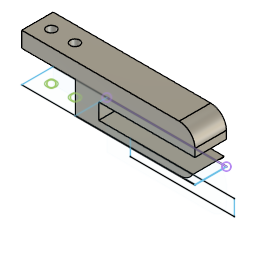
Boczniki (Autodesk Fusion 360 design; units mm, degrees)
part number: 2025-11-04-18-30-34-316
Autodesk Fusion 360 part; units mm, degrees
sketch "Szkic1" plane through (0, 0, 0) normal (0, 0, 1) x (1, 0, 0)
  line L0 (1, 16) -> (111, 16)
  line L1 (111, 16) -> (111, -4)
  line L2 (111, -4) -> (1, -4)
  line L3 (1, -4) -> (1, 16)
  line L4 (35.0688, 16) -> (111, 16)
  line L5 (111, 16) -> (111, -4)
  line L6 (111, -4) -> (35.0688, -4)
  line L7 (35.0688, -4) -> (35.0688, 16)
  circle A0 centre (9.8569, 6) radius 3
  circle A1 centre (24.8569, 6) radius 3
  dimension "d3" = 20
  dimension "d4" = 110
  dimension "d5" = 6
  dimension "d6" = 10
  dimension "d7" = 6
  constraint horizontal L0
  constraint vertical L1
  constraint horizontal L2
  constraint vertical L3
  constraint horizontal L4
  constraint vertical L5
  constraint horizontal L6
  constraint vertical L7
  constraint coincident L0 L4.start
  measures "d3" distance of L0.end L1.end
  measures "d4" distance of L0.start L0.end
  measures "d5" diameter of A0
  measures "d6" distance of L0 A0.centre
  measures "d7" diameter of A1
extrude "Wyciągnięcie proste1" add sketch "Szkic1" against normal blind 30 contours L0 L1 L2 L4 L5 L6 L7
extrude "Wyciągnięcie proste2" add sketch "Szkic1" against normal blind 10 contours L0 L2 L3 L7
fillet "Zaokrąglenie1" radius 10 1 edges at (111, 6, -30)
fillet "Zaokrąglenie2" radius 10 1 edges at (111, 6, 0)
sketch "Szkic2" plane through (0, 16, 0) normal (0, 1, 0) x (-1, 0, 0)
  arc A0 (-101, 0) -> (-111, -10) centre (-101, -10) ccw
  line L0 (-111, -10) -> (-111, -20)
  arc A1 (-111, -20) -> (-101, -30) centre (-101, -20) ccw
  line L1 (-101, -30) -> (-35.0688, -30)
  line L2 (-35.0688, -30) -> (-35.0688, -10)
  line L3 (-35.0688, -10) -> (-1, -10)
  line L4 (-1, -10) -> (-1, 0)
  line L5 (-1, 0) -> (-101, 0)
  line L6 (-35.0688, 0) -> (-111, 0)
  line L7 (-116, -15) -> (-50, -15)
  line L8 (-50, -15) -> (-50, -25)
  line L9 (-50, -25) -> (-116, -25)
  line L10 (-116, -25) -> (-116, -15)
  dimension "d18" = 5
  dimension "d19" = 10
  constraint horizontal L7
  constraint vertical L8
  constraint horizontal L9
  constraint vertical L10
  measures "d18" distance of L1 L9
  measures "d19" distance of L7 L9
extrude "Wyciągnięcie proste3" cut sketch "Szkic2" against normal blind 400 contours L0 A1 L7 L8 L9
move_body "Przesuń1" bodies 1 to x (1, 0, 0) y (0, 1, 0) z (0, 0, 1) at (0, 0, 30)
